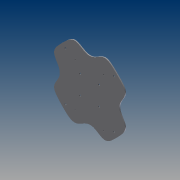
# Autodesk Inventor part: BaseTop
Saved by Autodesk Inventor 2011 SP1 (Build 150282100, 282)
## iProperties
Created: 2011-07-18
Part Number: BaseTop
Document SubType Name: Modeling
Designer: Nathan
Density: 1 g/cm^3
Author: Nathan
Autodesk Inventor part; units mm, degrees
ref_plane "YZ Plane" through (0, 0, 0) normal (1, 0, 0) x (0, 1, 0)
ref_plane "XZ Plane" through (0, 0, 0) normal (0, 1, 0) x (-1, 0, 0)
ref_plane "XY Plane" through (0, 0, 0) normal (0, 0, 1) x (1, 0, 0)
sketch "Sketch1" plane through (0, 0, 0) normal (0, 0, 1) x (1, 0, 0)
  line L0 (0, 3.1673) -> (0, -2.4908)
  line L1 (-20.5368, 0) -> (25.7294, 0)
  line L2 (0, 0) -> (-9.8402, -9.8402)
  line L3 (0, 0) -> (13.9161, 0) construction
  line L4 (0, 0) -> (-23.2805, 23.2805)
  spline S0 degree 5 poles (-23.2805, -60.3987) (-17.9127, -59.4483) (-8.7445, -53.5353) (6.2486, -38.505) (26.1605, -81.0323) (44.1438, -40.9875) (80.7734, -25.8575) (27.3972, 0.1894) (80.7453, 25.3359) (42.6686, 42.7055) (25.4142, 80.722) (0.0146, 27.4249) (-25.4543, 80.7206) (-42.5859, 42.7092) (-80.9328, 25.327) (-29.0929, 1.1966) (-78.7605, -24.9874) (-51.4868, -38.0314) (-37.726, -58.4925) (-28.7835, -61.373) (-23.2805, -60.3987) knots 0 0 0 0 0 0 0.074068 0.124068 0.186335 0.248602 0.311335 0.374068 0.436335 0.498602 0.561335 0.624068 0.686335 0.748602 0.811335 0.874068 0.924068 1 1 1 1 1 1
  point P0 (-16.1645, 16.1645)
  point P1 (-41.3092, 41.3092)
  point P2 (-41.3092, -41.3092)
  point P3 (-16.1645, -16.1645)
  point P4 (16.1645, 16.1645)
  point P5 (41.3092, 41.3092)
  point P6 (41.3092, -41.3092)
  point P7 (16.1645, -16.1645)
  point P8 (24.13, -47.9739)
  point P9 (24.13, 34.5761)
  point P10 (-24.13, 33.3061)
  point P11 (-24.13, -41.6239)
  point P12 (23.2805, -60.3987)
  point P13 (46.6973, -46.6973)
  point P14 (60.3987, -23.2805)
  point P15 (50.8, 0)
  point P16 (60.3987, 23.2805)
  point P17 (46.6973, 46.6973)
  point P18 (23.2805, 60.3987)
  point P19 (0, 50.8)
  point P20 (-23.2805, 60.3987)
  point P21 (-46.6973, 46.6973)
  point P22 (-60.3987, 23.2805)
  point P23 (-50.8, 0)
  point P24 (-60.3987, -23.2805)
  point P25 (-46.6973, -46.6973)
  dimension "d1" = 45
  dimension "d57" = 35.56
  dimension "d58" = 22.86
  dimension "d59" = 48.26
  dimension "d60" = 48.26
  dimension "d61" = 74.93
  dimension "d62" = 82.55
  dimension "d63" = 6.35
  dimension "d64" = 1.27
  dimension "d65" = 24.13
  constraints: 10 end point, 6 symmetric about line, 2 horizontal, 2 perpendicular, 2 point on line, 2 vertical, 1 equal length, 16 other
  measures "d1" angle of L3 L2
  measures "d57" distance of point (-41.309, 41.309) point (-16.164, 16.164)
  measures "d58" distance of L2.start point (-16.164, 16.164)
  measures "d59" horizontal distance of point (24.13, 34.576) point (-24.13, 33.306)
  measures "d60" horizontal distance of point (-24.13, -41.624) point (24.13, -47.974)
  measures "d61" distance of point (-24.13, -41.624) point (-24.13, 33.306)
  measures "d62" distance of point (24.13, 34.576) point (24.13, -47.974)
  measures "d63" vertical distance of point (-24.13, -41.624) point (24.13, -47.974)
  measures "d64" vertical distance of point (24.13, 34.576) point (-24.13, 33.306)
  measures "d65" distance from line of L0 point (-24.13, -41.624)
extrude "Extrusion1" add sketch "Sketch1" along normal blind 1.5875
hole "Hole1" at (-16.1645, 16.1645, 0) at (-41.3092, 41.3092, 0) at (-41.3092, -41.3092, 0) at (-16.1645, -16.1645, 0) at (41.3092, 41.3092, 0) at (16.1645, 16.1645, 0) at (16.1645, -16.1645, 0) at (41.3092, -41.3092, 0) direction (0, 0, 1) diameter 3.302 end through all thread size "8-32 UNC" class "2B" standard "ANSI Unified Screw Threads"
hole "Hole2" at (24.13, -47.9739, 0) at (24.13, 34.5761, 0) at (-24.13, 33.3061, 0) at (-24.13, -41.6239, 0) direction (0, 0, 1) diameter 2.159 end through all
body "Solid1"
